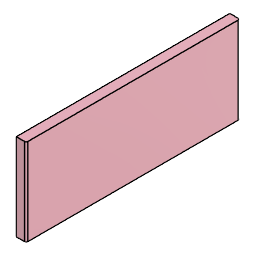
side_plate (Autodesk Fusion 360 design; units mm, degrees)
part number: 2025-10-03-12-31-24-970
Autodesk Fusion 360 part; units mm, degrees
sketch "Side Plate" plane through (0, 0, 0) normal (1, 0, 0) x (0, 1, 0)
  line L0 (0, 0) -> (256, 0)
  line L1 (256, 0) -> (256, 104)
  line L2 (256, 104) -> (0, 104)
  line L3 (0, 104) -> (0, 0)
  dimension "d4" = 104
  dimension "d5" = 256
  constraint horizontal L0
  constraint vertical L1
  constraint horizontal L2
  constraint vertical L3
  constraint coincident L0.start L3.end
  measures "d4" distance of L0.start L2.end
  measures "d5" distance of L0.start L0.end
extrude "Extrude1" add sketch "Side Plate" along normal blind 12
fillet "Fillet1" radius 2 2 edges at (12, 0, 52) (12, 256, 52)
equation "block_size = 16 mm" comment "The size of the blocks used for the dimensions of the Minecraft Pig."
equation "pine_thickness = 12 mm" comment "The thickness of the pine boards used for the Minecraft Pig's body."
equation "side_plate_height = 8 * block_size - 2 * pine_thickness" comment "The height of the Side Plates that make up the Minecraft Pig's body."
equation "d4 = side_plate_height"
equation "d5 = 16 * block_size"
equation "d6 = pine_thickness"
equation "fillet_radius = 2 mm" comment "The radius of the fillets applied to the Side Plates."
equation "d10 = fillet_radius"
named bodies: "Side Plate"
